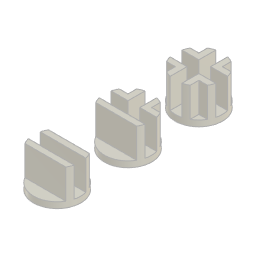
SourceFiles (Autodesk Fusion 360 design; units mm, degrees)
Autodesk Fusion 360 part; units mm, degrees
cylinder "CylinderPrimitive1" add diameter 40 height 30 placed x (1, 0, 0) y (0, 1, 0) z (0, 0, 1) at (0, 0, 0) makes body 1
box "BoxPrimitive1" cut length 10 width 40 height -25 placed x (0, 1, 0) y (-1, 0, 0) z (0, 0, 1) at (20, -5, 30) bodies 1
copy_body "CopyPasteBodies1" bodies 1 makes body 2
move_body "Move1" bodies 2 to x (1, 0, 0) y (0, 1, 0) z (0, 0, 1) at (0, 60, 0)
box "BoxPrimitive2" cut length 20 width 10 height -25 placed x (0, 1, 0) y (-1, 0, 0) z (0, 0, 1) at (5, 65, 30) bodies 2
copy_body "CopyPasteBodies2" bodies 2 makes body 3
move_body "Move2" bodies 3 to x (1, 0, 0) y (0, 1, 0) z (0, 0, 1) at (0, 60, 0)
box "BoxPrimitive3" cut length 11 width 40 height -25 placed x (0, 1, 0) y (-1, 0, 0) z (0, 0, 1) at (20, -21, 30) bodies 1
box "BoxPrimitive4" cut length 12 width 40 height -25 placed x (0, 1, 0) y (-1, 0, 0) z (0, 0, 1) at (20, 10, 30) bodies 1
box "BoxPrimitive5" cut length 10 width 10 height -25 placed x (0, 1, 0) y (-1, 0, 0) z (0, 0, 1) at (20, 70, 30) bodies 2
box "BoxPrimitive6" cut length 10 width 10 height -25 placed x (0, 1, 0) y (-1, 0, 0) z (0, 0, 1) at (-10, 70, 30) bodies 2
box "BoxPrimitive7" cut length 11 width 40 height -25 placed x (0, 1, 0) y (-1, 0, 0) z (0, 0, 1) at (20, 39, 30) bodies 2
box "BoxPrimitive8" cut length 20 width 10 height -25 placed x (0, -1, 0) y (1, 0, 0) z (0, 0, 1) at (-5, 115, 30) bodies 3
box "BoxPrimitive9" cut length 10 width 10 height -25 placed x (0, -1, 0) y (1, 0, 0) z (0, 0, 1) at (-20, 140, 30) bodies 3
box "BoxPrimitive10" cut length 15 width 15 height -25 placed x (0, -1, 0) y (1, 0, 0) z (0, 0, 1) at (-25, 110, 30) bodies 3
box "BoxPrimitive11" cut length 10 width 10 height -25 placed x (0, -1, 0) y (1, 0, 0) z (0, 0, 1) at (10, 110, 30) bodies 3
box "BoxPrimitive12" cut length 20 width 15 height -25 placed x (0, 1, 0) y (-1, 0, 0) z (0, 0, 1) at (25, 130, 30) bodies 3
named bodies: "I Joint", "T Joint", "Plus Joint"
